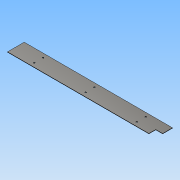
# Autodesk Inventor part: Leistenbürstenblech
Saved by Autodesk Inventor 2019.4 (Build 234330000, 330)
## iProperties
Created: 2017-11-30
Part Number: Leistenbürstenblech
Material: 1.4301
Document SubType Name: Sheet Metal
Designer: ees GmbH
Density: 7.9 g/cm^3
Sheet Metal Rule: Standard_mm
Appearance: Halbpoliert(5)
Mass: 3230.34 g
Surface Area: 4125.84 cm^2
Volume: 1196.42 cm^3
Flat Pattern Width: 75.2 cm
Flat Pattern Length: 8.5 cm
Flat Pattern Area: 639.2 cm^2
Sheet Metal Width: 752,000 mm
Sheet Metal Length: 85,000 mm
Sheet Metal Area: 63920,000 mm^2
Description: Leistenbürstenblech
Stock Number: 2007.003-00.00-012
Masse: 1.26 kg
Blechmasse: 195 mm x 400 mm x 6 mm
Abmessung: =Bl <Stärke>
Stärke: 1,5
Author: ees GmbH
Autodesk Inventor part; units mm, degrees
ref_plane "YZ Plane" through (0, 0, 0) normal (1, 0, 0) x (0, 1, 0)
ref_plane "XZ Plane" through (0, 0, 0) normal (0, 1, 0) x (-1, 0, 0)
ref_plane "XY Plane" through (0, 0, 0) normal (0, 0, 1) x (1, 0, 0)
derived "Parameter Skizze.ipt"
sketch "Skizze5" plane through (0, 0, 0) normal (0, 0, 1) x (1, 0, 0)
  line L0 (-376, 42.5) -> (376, 42.5)
  line L1 (376, 42.5) -> (376, -42.5)
  line L2 (376, -42.5) -> (-376, -42.5)
  line L3 (-376, -42.5) -> (-376, 42.5)
  point P0 (0, 0)
  point P1 (0, 42.5)
  point P2 (-376, 0)
  dimension "d1" = 752
  dimension "d2" = 85
  measures "d1" distance of L0.start L0.end
  measures "d2" distance of L2.end L0.start
extrude "Grobblech1" add sketch "Skizze5" along normal blind 1.5
sketch "Skizze1" plane through (0, 0, 0) normal (0, 1, 0) x (-1, 0, 0)
  line L0 (1120, 528.75) -> (-1120, 528.75)
  line L1 (-1120, 528.75) -> (-1120, -528.75)
  line L2 (-1120, -528.75) -> (1120, -528.75)
  line L3 (1120, -528.75) -> (1120, 528.75)
  line L4 (1120, -243.75) -> (-1120, -243.75)
  line L5 (-924, -243.75) -> (-924, -528.75)
  point P0 (0, 0)
  point P1 (-1120, 0)
  point P2 (0, 528.75)
  point P3 (0, -528.75)
sketch "Skizze2" plane through (0, 0, 0) normal (0, 0, 1) x (1, 0, 0)
  line L0 (-895.5, 600) -> (895.5, 600)
  line L1 (1120, 375.5) -> (1120, -375.5)
  line L2 (895.5, -600) -> (-895.5, -600)
  line L3 (-1120, -375.5) -> (-1120, 375.5)
  arc A0 (895.5, -600) -> (1120, -375.5) centre (895.5, -375.5) ccw
  arc A1 (-1120, -375.5) -> (-895.5, -600) centre (-895.5, -375.5) ccw
  arc A2 (1120, 375.5) -> (895.5, 600) centre (895.5, 375.5) ccw
  arc A3 (-895.5, 600) -> (-1120, 375.5) centre (-895.5, 375.5) ccw
  point P0 (0, 0)
  point P1 (-1120, 600)
  point P2 (-1120, -600)
  point P3 (-1120, 0)
  point P4 (-1120, 0)
  point P5 (-1120, 0)
  point P6 (1120, 0)
  point P7 (1120, 0)
  point P8 (1120, 0)
  point P9 (1120, 0)
sketch "Skizze3" plane through (0, 0, 0) normal (1, 0, 0) x (0, 1, 0)
  line L0 (600, 528.75) -> (-600, 528.75)
  line L1 (-600, 528.75) -> (-600, -528.75)
  line L2 (-600, -528.75) -> (600, -528.75)
  line L3 (600, -528.75) -> (600, 528.75)
  line L4 (-320, 528.75) -> (320, 528.75)
  line L5 (320, 528.75) -> (320, -528.75)
  line L6 (320, -528.75) -> (-320, -528.75)
  line L7 (-320, -528.75) -> (-320, 528.75)
  line L8 (-600, 0) -> (600, 0)
  line L9 (0, -528.75) -> (0, 528.75)
  line L10 (-375.5, 0) -> (-600, 0)
  line L11 (320, -233.75) -> (600, -209.2532)
  point P0 (0, 0)
  point P1 (0, -243.75)
  point P2 (0, -243.75)
  point P3 (0, -243.75)
sketch "Skizze6" plane through (0, 0, 1.5) normal (0, 0, 1) x (1, 0, 0)
  line L0 (-260, 22.5) -> (-260, 0)
  line L1 (-260, 0) -> (-260, -22.5) construction
  line L2 (-376, -42.5) -> (-376, 42.5) projected
  line L3 (-260, 22.5) -> (260, 22.5) construction
  line L4 (260, 22.5) -> (260, -22.5)
  line L5 (260, -22.5) -> (-260, -22.5) construction
  line L6 (-376, 42.5) -> (376, 42.5) projected
  line L7 (-376, 42.5) -> (376, 42.5) projected
  line L8 (376, -42.5) -> (-376, -42.5) projected
  line L9 (0, 22.5) -> (0, -22.5)
  point P0 (0, 0)
  point P1 (0, 0)
  point P2 (-376, 0)
  point P3 (-376, 0)
  dimension "d13" = 45
  dimension "d14" = 116
  dimension "d36" = 520
  dimension "d40" = 20
  constraints: 13 end point, 4 midpoint, 3 vertical, 2 coincident, 2 horizontal, 1 collinear, 1 horizontal alignment
  measures "d13" distance of L1.end L0.start
  measures "d14" distance between parallel lines of L2 L0
  measures "d36" distance of L0.start L3.end
  measures "d40" distance from line of L0.start L6
hole "Bohrung1" at (-260, 22.5, 1.5) at (-260, -22.5, 1.5) at (0, 22.5, 1.5) at (0, -22.5, 1.5) at (260, 22.5, 1.5) at (260, -22.5, 1.5) direction (0, 0, -1) diameter 6.6 end through all clearance for "Sechskantkopfschraube DIN EN 24017" size "M6" standard "DIN"
sketch "Skizze11" plane through (0, 0, 1.5) normal (0, 0, 1) x (1, 0, 0)
  line L0 (-376, 42.5) -> (376, 42.5) projected
  line L1 (376, -42.5) -> (-376, -42.5) projected
  line L2 (376, -42.5) -> (341, -42.5)
  line L3 (341, -42.5) -> (341, -7.5)
  line L4 (341, -7.5) -> (376, -7.5)
  line L5 (376, -7.5) -> (376, -42.5)
  point P0 (0, 0)
  dimension "d81" = 35
  dimension "d82" = 35
  constraints: 8 end point, 2 parallel, 1 horizontal, 1 perpendicular
  measures "d81" distance of L3.end L4.end
  measures "d82" distance of L4.end L1.start
extrude "Ausklinkung1" cut sketch "Skizze11" against normal blind 1.5
equation "\"d11\" = Stärke"
equation "\"d79\" = Stärke"
equation "\"d44\" = Stärke"
equation "\"Biegeradius\" = Stärke"
equation "\"BreiteBiegungsfreistellung\" = Stärke"
equation "\"TiefeBiegungsfreistellung\" = 0.5 * Stärke"
equation "\"GrößeEckenfreistellung\" = 4 * Stärke"
equation "\"MinimalRest\" = 2 * Stärke"
equation "\"Übergangsradius\" = Biegeradius"
equation "\"JacobiRadiusGröße\" = Biegeradius"
equation "\"Abstandsgröße\" = Stärke"
equation "\"d3\" = Biegeradius"
equation "\"Stärke\" = 1.5"
